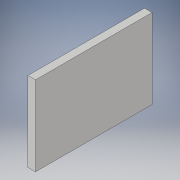
# Autodesk Inventor part: Part2
Saved by Autodesk Inventor 2019 (Build 230136000, 136)
## iProperties
Created: 2019-12-09
Part Number: Part2
Material: Generic
Document SubType Name: Modeling
Designer: ABHISHEK
Density: 1 g/cm^3
Appearance: Default
Author: ABHISHEK
Autodesk Inventor part; units mm, degrees
ref_plane "YZ Plane" through (0, 0, 0) normal (1, 0, 0) x (0, 1, 0)
ref_plane "XZ Plane" through (0, 0, 0) normal (0, 1, 0) x (-1, 0, 0)
ref_plane "XY Plane" through (0, 0, 0) normal (0, 0, 1) x (1, 0, 0)
sketch "Sketch1" plane through (0, 0, 0) normal (1, 0, 0) x (0, 1, 0)
  line L0 (5.8895, 108.115) -> (-78.3115, 108.115)
  line L1 (-78.3115, 108.115) -> (-78.3115, -15.1258)
  line L2 (-78.3115, -15.1258) -> (5.8895, -15.1258)
  line L3 (5.8895, -15.1258) -> (5.8895, 108.115)
  point P0 (0, 0)
  dimension "d0" = 84.201
  dimension "d1" = 123.2408
  constraints: 8 end point, 2 parallel, 1 horizontal, 1 perpendicular
  measures "d0" distance of L2.end L1.end
  measures "d1" distance between parallel lines of L2 L0
extrude "Extrusion1" add sketch "Sketch1" along normal blind 8
body "Solid1"
